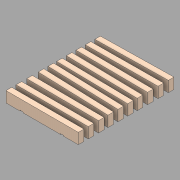
# Autodesk Inventor part: dormente_final
Saved by Autodesk Inventor 2018 (Build 220112000, 112)
## iProperties
Created: 2018-08-09
Part Number: dormente_final
Material: Wood (Birch)
Document SubType Name: Modeling
Designer: flavi
Density: 0.55 g/cm^3
Appearance: Birch - Natural Polished
Mass: 79200 g
Surface Area: 23040 cm^2
Volume: 144000 cm^3
Author: flavi
Autodesk Inventor part; units mm, degrees
ref_plane "YZ Plane" through (0, 0, 0) normal (1, 0, 0) x (0, 1, 0)
ref_plane "XZ Plane" through (0, 0, 0) normal (0, 1, 0) x (-1, 0, 0)
ref_plane "XY Plane" through (0, 0, 0) normal (0, 0, 1) x (1, 0, 0)
sketch "Sketch5" plane through (0, 0, 0) normal (0, 0, 1) x (1, 0, 0)
  line L0 (-20730, -264417.3398) -> (-20730, -262313.5359)
  line L1 (-20730, -260695.3081) -> (-20730, -258591.5042)
  line L2 (-20730, -256710.4016) -> (-20730, -254606.5977)
  line L3 (-20730, -252422.8748) -> (-20730, -250319.0709)
  line L4 (-20730, -248750.3548) -> (-20730, -246646.5509)
  line L5 (-20730, -241909.1189) -> (-20730, -239805.315)
  line L6 (-20730, -238349.0223) -> (-20730, -236245.2184)
  line L7 (-20730, -234866.3859) -> (-20730, -232762.582)
  line L8 (-20730, -231302.8852) -> (-20730, -229199.0813)
  line L9 (-20730, -243453.9106) -> (-20730, -245557.7145)
  line L10 (6242.9418, -264417.3398) -> (6242.9418, -262313.5359)
  line L11 (6242.9412, -260720.3148) -> (6242.9412, -258616.5109)
  line L12 (6242.9412, -256890.9666) -> (6242.9412, -254787.1627)
  line L13 (6242.9412, -253363.9723) -> (6242.9412, -251260.1684)
  line L14 (6242.9412, -249623.3537) -> (6242.9412, -247519.5498)
  line L15 (6242.9412, -246003.92) -> (6242.9412, -243900.1161)
  line L16 (6242.9412, -242439.6002) -> (6242.9412, -240335.7963)
  line L17 (6242.9412, -238586.3047) -> (6242.9412, -236482.5008)
  line L18 (6242.9412, -234655.2907) -> (6242.9412, -232551.4868)
  line L19 (6242.9412, -230805.0616) -> (6242.9412, -228701.2577)
  line L20 (6242.9418, -264417.3398) -> (-20730, -264417.3398)
  line L21 (-20730, -262313.5359) -> (6242.9418, -262313.5359)
  line L22 (6242.9412, -260720.3148) -> (-20730, -260695.3081)
  line L23 (-20730, -258591.5042) -> (6242.9412, -258616.5109)
  line L24 (6242.9412, -256890.9666) -> (-20730, -256710.4016)
  line L25 (-20730, -254606.5977) -> (6242.9412, -254787.1627)
  line L26 (6242.9412, -253363.9723) -> (-20730, -252422.8748)
  line L27 (-20730, -250319.0709) -> (6242.9412, -251260.1684)
  line L28 (6242.9412, -249623.3537) -> (-20730, -248750.3548)
  line L29 (-20730, -246646.5509) -> (6242.9412, -247519.5498)
  line L30 (6242.9412, -246003.92) -> (-20730, -245557.7145)
  line L31 (-20730, -243453.9106) -> (6242.9412, -243900.1161)
  line L32 (-20730, -241909.1189) -> (6242.9412, -242439.6002)
  line L33 (6242.9412, -240335.7963) -> (-20730, -239805.315)
  line L34 (-20730, -238349.0223) -> (6242.9412, -238586.3047)
  line L35 (6242.9412, -236482.5008) -> (-20730, -236245.2184)
  line L36 (-20730, -234866.3859) -> (6242.9412, -234655.2907)
  line L37 (6242.9412, -232551.4868) -> (-20730, -232762.582)
  line L38 (-20730, -231302.8852) -> (6242.9412, -230805.0616)
  line L39 (6242.9412, -228701.2577) -> (-20730, -229199.0813)
  point P0 (0, 0)
  point P1 (-20967.6471, -21622.2237)
  point P2 (6005.2941, -22128.6389)
  point P3 (-20967.6471, -23726.0276)
  point P4 (6005.2941, -24232.4428)
  point P5 (-20967.6471, -25741.5078)
  point P6 (6005.2941, -26024.2617)
  point P7 (-20967.6471, -27845.3117)
  point P8 (6005.2941, -28128.0656)
  point P9 (-20967.6471, -29322.81)
  point P10 (6005.2941, -29455.9796)
  point P11 (-20967.6471, -31426.6139)
  point P12 (6005.2941, -31559.7835)
  point P13 (-20967.6471, -32751.5457)
  point P14 (6005.2941, -33039.4294)
  point P15 (-20967.6471, -34855.3496)
  point P16 (6005.2941, -35143.2333)
  point P17 (-20967.6471, -36586.2217)
  point P18 (6005.2941, -36019.7541)
  point P19 (-20967.6471, -38690.0256)
  point P20 (6005.2941, -38123.558)
  point P21 (-20967.6471, -40394.1013)
  point P22 (6005.2941, -39825.798)
  point P23 (-20967.6471, -42497.9052)
  point P24 (6005.2941, -41929.6019)
  point P25 (-20967.6471, -44164.6545)
  point P26 (6005.2941, -43868.5054)
  point P27 (-20967.6471, -46268.4584)
  point P28 (6005.2941, -45972.3094)
  point P29 (-20967.6471, -47624.7575)
  point P30 (6124.1176, -47419.887)
  point P31 (-20967.6471, -49728.5614)
  point P32 (6124.1176, -49523.6909)
  point P33 (-20967.6471, -51405.068)
  point P34 (6124.1176, -50852.6184)
  point P35 (-20967.6471, -53508.8719)
  point P36 (6124.1176, -52956.4223)
  point P37 (-20967.6471, -58361.4939)
  point P38 (6124.1176, -57120.5712)
  point P39 (-20967.6471, -60465.2978)
  point P40 (6124.1176, -59224.3751)
  point P41 (-20967.6471, -60920.5609)
  point P42 (6124.1176, -60371.9053)
  point P43 (-20967.6471, -63024.3648)
  point P44 (6124.1176, -62475.7093)
  point P45 (-20848.8235, -64155.5217)
  point P46 (6124.1176, -64350.4137)
  point P47 (-20848.8235, -66259.3256)
  point P48 (6124.1176, -66454.2176)
  point P49 (-20848.8235, -67844.0876)
  point P50 (6124.1176, -68075.3244)
  point P51 (-20848.8235, -69947.8915)
  point P52 (6124.1176, -70179.1283)
  point P53 (-20848.8235, -71566.6692)
  point P54 (6124.1176, -71765.9876)
  point P55 (-20848.8235, -73670.4731)
  point P56 (6124.1176, -73869.7915)
  point P57 (-20848.8235, -75189.4885)
  point P58 (6124.1176, -75557.0021)
  point P59 (-20848.8235, -77293.2924)
  point P60 (6124.1176, -77660.806)
  point P61 (-20848.8235, -78800.4247)
  point P62 (6124.1176, -79158.9919)
  point P63 (-20848.8235, -80904.2286)
  point P64 (6124.1176, -81262.7958)
  point P65 (-20848.8235, -82340.3345)
  point P66 (6124.1176, -82631.5147)
  point P67 (-20848.8235, -84444.1384)
  point P68 (6124.1176, -84735.3186)
  point P69 (-20848.8235, -86304.7162)
  point P70 (6124.1176, -85878.5865)
  point P71 (-20848.8235, -88408.5201)
  point P72 (6124.1176, -87982.3904)
  point P73 (-20848.8235, -89831.6613)
  point P74 (6124.1176, -90167.2876)
  point P75 (-20848.8235, -91935.4652)
  point P76 (6124.1176, -92271.0915)
  point P77 (-20848.8235, -93513.8337)
  point P78 (6124.1176, -93898.5101)
  point P79 (-20848.8235, -95617.6376)
  point P80 (6124.1176, -96002.314)
  point P81 (-20848.8235, -102847.812)
  point P82 (6124.1176, -102395.7335)
  point P83 (-20848.8235, -104951.6159)
  point P84 (6124.1176, -104499.5374)
  point P85 (-20848.8235, -106342.4532)
  point P86 (6124.1176, -106515.4114)
  point P87 (-20848.8235, -108446.2571)
  point P88 (6124.1176, -108619.2153)
  point P89 (-20848.8235, -109981.1716)
  point P90 (6124.1176, -110089.6631)
  point P91 (-20848.8235, -112084.9755)
  point P92 (6124.1176, -112193.467)
  point P93 (-20848.8235, -113751.8742)
  point P94 (6124.1176, -113732.3134)
  point P95 (-20848.8235, -115855.6781)
  point P96 (6124.1176, -115836.1173)
  point P97 (-20848.8235, -117298.3112)
  point P98 (6124.1176, -117799.6039)
  point P99 (-20848.8235, -119402.1151)
  point P100 (6124.1176, -119903.4078)
  point P101 (-20848.8235, -120988.6147)
  point P102 (6124.1176, -121322.2726)
  point P103 (-20848.8235, -123092.4186)
  point P104 (6124.1176, -123426.0765)
  point P105 (-20848.8235, -124104.6291)
  point P106 (6124.1176, -124617.6757)
  point P107 (-20848.8235, -126208.433)
  point P108 (6124.1176, -126721.4796)
  point P109 (-20848.8235, -127960.9362)
  point P110 (6124.1176, -128375.0805)
  point P111 (-20848.8235, -130064.7401)
  point P112 (6124.1176, -130478.8844)
  point P113 (-20848.8235, -132255.5715)
  point P114 (6124.1176, -132095.4557)
  point P115 (-20848.8235, -134359.3754)
  point P116 (6124.1176, -134199.2597)
  point P117 (-20848.8235, -135675.5926)
  point P118 (6124.1176, -135487.8273)
  point P119 (-20848.8235, -137779.3965)
  point P120 (6124.1176, -137591.6312)
  point P121 (-20848.8235, -144607.9861)
  point P122 (6124.1176, -144387.8571)
  point P123 (-20848.8235, -146711.79)
  point P124 (6124.1176, -146491.661)
  point P125 (-20848.8235, -148314.0751)
  point P126 (6124.1176, -148295.1438)
  point P127 (-20848.8235, -150417.879)
  point P128 (6124.1176, -150398.9477)
  point P129 (-20848.8235, -152139.9424)
  point P130 (6124.1176, -152482.8636)
  point P131 (-20848.8235, -154243.7463)
  point P132 (6124.1176, -154586.6675)
  point P133 (-20848.8235, -155757.3569)
  point P134 (6124.1176, -156278.2711)
  point P135 (-20848.8235, -157861.1608)
  point P136 (6124.1176, -158382.075)
  point P137 (-20848.8235, -159323.05)
  point P138 (6124.1176, -159925.243)
  point P139 (-20848.8235, -161426.8539)
  point P140 (6124.1176, -162029.0469)
  point P141 (-20848.8235, -162986.1529)
  point P142 (6124.1176, -163475.4003)
  point P143 (-20848.8235, -165089.9568)
  point P144 (6124.1176, -165579.2042)
  point P145 (-20848.8235, -166721.6427)
  point P146 (6124.1176, -167153.3914)
  point P147 (-20848.8235, -168825.4466)
  point P148 (6124.1176, -169257.1953)
  point P149 (-20848.8235, -170217.6991)
  point P150 (6242.9412, -170671.8236)
  point P151 (-20848.8235, -172321.503)
  point P152 (6242.9412, -172775.6275)
  point P153 (-20848.8235, -174234.1043)
  point P154 (6242.9412, -174268.9144)
  point P155 (-20848.8235, -176337.9082)
  point P156 (6242.9412, -176372.7184)
  point P157 (-20848.8235, -178049.9898)
  point P158 (6242.9412, -177866.4022)
  point P159 (-20848.8235, -180153.7937)
  point P160 (6242.9412, -179970.2061)
  point P161 (-20848.8235, -186925.1382)
  point P162 (6242.9412, -187023.8253)
  point P163 (-20848.8235, -189028.9421)
  point P164 (6242.9412, -189127.6292)
  point P165 (-20730, -190608.4103)
  point P166 (6242.9412, -190955.6253)
  point P167 (-20730, -192712.2142)
  point P168 (6242.9412, -193059.4292)
  point P169 (-20730, -194360.1448)
  point P170 (6242.9412, -194817.9349)
  point P171 (-20730, -196463.9487)
  point P172 (6242.9412, -196921.7388)
  point P173 (-20730, -198017.5791)
  point P174 (6242.9412, -198574.0909)
  point P175 (-20730, -200121.383)
  point P176 (6242.9412, -200677.8948)
  point P177 (-20730, -201788.5309)
  point P178 (6242.9412, -202216.0346)
  point P179 (-20730, -203892.3348)
  point P180 (6242.9412, -204319.8385)
  point P181 (-20730, -205635.6546)
  point P182 (6242.9412, -205781.4811)
  point P183 (-20730, -207739.4585)
  point P184 (6242.9412, -207885.285)
  point P185 (-20730, -209497.3663)
  point P186 (6242.9412, -209131.5896)
  point P187 (-20730, -211601.1702)
  point P188 (6242.9412, -211235.3935)
  point P189 (-20730, -213181.738)
  point P190 (6242.9412, -212258.4637)
  point P191 (-20730, -215285.5419)
  point P192 (6242.9412, -214362.2676)
  point P193 (-20730, -216668.1961)
  point P194 (6242.9412, -215985.7199)
  point P195 (-20730, -218772)
  point P196 (6242.9412, -218089.5238)
  point P197 (-20730, -220095.541)
  point P198 (6242.9412, -219772.1543)
  point P199 (-20730, -222199.3449)
  constraints: 80 end point, 10 parallel, 3 vertical, 1 horizontal
sketch "Sketch6" plane through (0, 0, 0) normal (0, 0, 1) x (1, 0, 0)
  line L0 (-411.1765, -264436.5073) -> (-411.1765, -262309.305)
  line L1 (-411.1765, -262309.305) -> (-411.1765, -260714.1457)
  line L2 (-411.1765, -260714.1457) -> (-411.1765, -258610.3418)
  line L3 (-411.1765, -258610.3418) -> (-411.1765, -256846.4219)
  line L4 (-411.1765, -256846.4219) -> (-411.1765, -254742.618)
  line L5 (-411.1765, -254742.618) -> (-292.3529, -253135.9531)
  line L6 (-292.3529, -253135.9531) -> (-292.3529, -251032.1492)
  line L7 (-292.3529, -251032.1492) -> (-292.3529, -249411.8341)
  line L8 (-292.3529, -249411.8341) -> (-292.3529, -247308.0302)
  line L9 (-292.3529, -247308.0302) -> (-292.3529, -245895.8085)
  line L10 (-292.3529, -245895.8085) -> (-292.3529, -243792.0046)
  line L11 (-292.3529, -243792.0046) -> (-411.1765, -242308.7326)
  line L12 (-411.1765, -242308.7326) -> (-411.1765, -240204.9286)
  line L13 (-411.1765, -240204.9286) -> (-411.1765, -238527.7681)
  line L14 (-411.1765, -238527.7681) -> (-411.1765, -236423.9642)
  line L15 (-411.1765, -236423.9642) -> (-411.1765, -234707.3671)
  line L16 (-411.1765, -234707.3671) -> (-411.1765, -232603.5631)
  line L17 (-411.1765, -232603.5631) -> (-287.1139, -230926.0589)
  line L18 (-287.1139, -230926.0589) -> (-287.1139, -228740.268)
  line L19 (-287.1139, -228740.268) -> (777.2418, -228740.268)
  line L20 (777.2418, -228740.268) -> (777.2418, -230906.1896)
  line L21 (777.2418, -230906.1896) -> (777.2418, -232594.5112)
  line L22 (777.2418, -232594.5112) -> (777.2418, -234698.3151)
  line L23 (777.2418, -234698.3151) -> (777.2418, -236434.6646)
  line L24 (777.2418, -236434.6646) -> (777.2418, -238538.4685)
  line L25 (777.2418, -238538.4685) -> (777.2418, -240228.5453)
  line L26 (777.2418, -240228.5453) -> (777.2418, -242332.3492)
  line L27 (777.2418, -242332.3492) -> (777.2418, -243809.943)
  line L28 (777.2418, -243809.943) -> (777.2418, -245913.7469)
  line L29 (777.2418, -245913.7469) -> (777.2418, -247342.8899)
  line L30 (777.2418, -247342.8899) -> (777.2418, -249446.6938)
  line L31 (777.2418, -249446.6938) -> (777.2418, -251069.7089)
  line L32 (777.2418, -251069.7089) -> (777.2418, -253173.5128)
  line L33 (777.2418, -253173.5128) -> (777.2418, -254750.8199)
  line L34 (777.2418, -254750.8199) -> (777.2418, -256854.6238)
  line L35 (777.2418, -256854.6238) -> (777.2418, -258611.6909)
  line L36 (777.2418, -258611.6909) -> (777.2418, -260715.4948)
  line L37 (777.2418, -260715.4948) -> (777.2418, -262309.305)
  line L38 (777.2418, -262309.305) -> (777.2418, -264436.5073)
  line L39 (777.2418, -264436.5073) -> (-411.1765, -264436.5073)
  line L40 (-14313.5294, -264431.9833) -> (-14313.5294, -262312.3235)
  line L41 (-14313.5294, -262312.3235) -> (-14313.5294, -260701.3806)
  line L42 (-14313.5294, -260701.3806) -> (-14313.5294, -258597.5767)
  line L43 (-14313.5294, -258597.5767) -> (-14313.5294, -256753.4791)
  line L44 (-14313.5294, -256753.4791) -> (-14313.5294, -254649.6752)
  line L45 (-14313.5294, -254649.6752) -> (-14313.5294, -252646.872)
  line L46 (-14313.5294, -252646.872) -> (-14313.5294, -250543.068)
  line L47 (-14313.5294, -250543.068) -> (-14313.5294, -248958.1522)
  line L48 (-14313.5294, -248958.1522) -> (-14313.5294, -246854.3483)
  line L49 (-14313.5294, -246854.3483) -> (-14313.5294, -245663.984)
  line L50 (-14313.5294, -245663.984) -> (-14313.5294, -243560.1801)
  line L51 (-14313.5294, -243560.1801) -> (-14313.5294, -229054.1614)
  line L52 (-14313.5294, -229054.1614) -> (-15501.7647, -229075.8446)
  line L53 (-15501.7647, -229075.8446) -> (-15501.7647, -231206.2671)
  line L54 (-15501.7647, -231206.2671) -> (-15501.7647, -232721.5412)
  line L55 (-15501.7647, -232721.5412) -> (-15501.7647, -260700.0315)
  line L56 (-15501.7647, -260700.0315) -> (-15501.7647, -262312.3235)
  line L57 (-15501.7647, -262312.3235) -> (-15501.7647, -264431.9833)
  line L58 (-15501.7647, -264431.9833) -> (-14313.5294, -264431.9833)
  point P0 (0, 0)
  point P1 (-15739.4118, -21720.3835)
  point P2 (-14551.1765, -21742.6925)
  point P3 (-411.1765, -22008.1701)
  point P4 (777.0588, -22030.4791)
  point P5 (-15739.4118, -23824.1874)
  point P6 (-14551.1765, -23846.4964)
  point P7 (-411.1765, -24111.974)
  point P8 (777.0588, -24134.283)
  point P9 (-15739.4118, -25796.3147)
  point P10 (-14551.1765, -25808.7709)
  point P11 (-411.1765, -25956.9987)
  point P12 (777.0588, -25969.4548)
  point P13 (-15739.4118, -27900.1186)
  point P14 (-14551.1765, -27912.5748)
  point P15 (-411.1765, -28060.8026)
  point P16 (777.0588, -28073.2587)
  point P17 (-15739.4118, -29348.6226)
  point P18 (-14551.1765, -29354.4891)
  point P19 (-411.1765, -29424.3005)
  point P20 (777.0588, -29430.167)
  point P21 (-15739.4118, -31452.4265)
  point P22 (-14551.1765, -31458.293)
  point P23 (-411.1765, -31528.1044)
  point P24 (777.0588, -31533.9709)
  point P25 (-15739.4118, -32807.347)
  point P26 (-14551.1765, -32820.0291)
  point P27 (-411.1765, -32970.9461)
  point P28 (777.0588, -32983.6282)
  point P29 (-15739.4118, -34911.1509)
  point P30 (-14551.1765, -34923.833)
  point P31 (-411.1765, -35074.75)
  point P32 (777.0588, -35087.4321)
  point P33 (-15739.4118, -36476.4218)
  point P34 (-14551.1765, -36451.4673)
  point P35 (-411.1765, -36154.5085)
  point P36 (777.0588, -36129.554)
  point P37 (-15739.4118, -38580.2257)
  point P38 (-14551.1765, -38555.2712)
  point P39 (-411.1765, -38258.3124)
  point P40 (777.0588, -38233.3579)
  point P41 (-15739.4118, -40283.9456)
  point P42 (-14551.1765, -40258.9102)
  point P43 (-411.1765, -39960.9891)
  point P44 (777.0588, -39935.9537)
  point P45 (-15739.4118, -42387.7495)
  point P46 (-14551.1765, -42362.7141)
  point P47 (-411.1765, -42064.793)
  point P48 (777.0588, -42039.7576)
  point P49 (-15739.4118, -44107.2512)
  point P50 (-14551.1765, -44094.205)
  point P51 (-411.1765, -43938.955)
  point P52 (777.0588, -43925.9088)
  point P53 (-15739.4118, -46211.0551)
  point P54 (-14551.1765, -46198.0089)
  point P55 (-411.1765, -46042.7589)
  point P56 (777.0588, -46029.7127)
  point P57 (-15739.4118, -47585.2211)
  point P58 (-14551.1765, -47576.2356)
  point P59 (-411.1765, -47469.3075)
  point P60 (777.0588, -47460.3219)
  point P61 (-15739.4118, -49689.025)
  point P62 (-14551.1765, -49680.0395)
  point P63 (-411.1765, -49573.1114)
  point P64 (777.0588, -49564.1259)
  point P65 (-15739.4118, -51298.4549)
  point P66 (-14551.1765, -51274.2246)
  point P67 (-411.1765, -50985.8847)
  point P68 (777.0588, -50961.6545)
  point P69 (-15739.4118, -53402.2588)
  point P70 (-14551.1765, -53378.0285)
  point P71 (-411.1765, -53089.6886)
  point P72 (777.0588, -53065.4584)
  point P73 (-15739.4118, -58122.0176)
  point P74 (-14551.1765, -58067.5912)
  point P75 (-292.3529, -57414.4739)
  point P76 (777.0588, -57365.4901)
  point P77 (-15739.4118, -60225.8215)
  point P78 (-14551.1765, -60171.3951)
  point P79 (-292.3529, -59518.2778)
  point P80 (777.0588, -59469.294)
  point P81 (-15739.4118, -60814.68)
  point P82 (-14551.1765, -60790.6162)
  point P83 (-411.1765, -60504.2565)
  point P84 (777.0588, -60480.1926)
  point P85 (-15739.4118, -62918.4839)
  point P86 (-14551.1765, -62894.4201)
  point P87 (-411.1765, -62608.0604)
  point P88 (777.0588, -62583.9965)
  point P89 (-15739.4118, -64192.4395)
  point P90 (-14551.1765, -64201.0251)
  point P91 (-411.1765, -64303.1932)
  point P92 (777.0588, -64311.7787)
  point P93 (-15739.4118, -66296.2434)
  point P94 (-14551.1765, -66304.829)
  point P95 (-411.1765, -66406.9971)
  point P96 (777.0588, -66415.5826)
  point P97 (-15739.4118, -67887.8901)
  point P98 (-14551.1765, -67898.0768)
  point P99 (-411.1765, -68019.2978)
  point P100 (777.0588, -68029.4845)
  point P101 (-15739.4118, -69991.6941)
  point P102 (-14551.1765, -70001.8807)
  point P103 (-411.1765, -70123.1017)
  point P104 (777.0588, -70133.2884)
  point P105 (-15739.4118, -71604.4255)
  point P106 (-14551.1765, -71613.2061)
  point P107 (-411.1765, -71717.6946)
  point P108 (777.0588, -71726.4751)
  point P109 (-15739.4118, -73708.2295)
  point P110 (-14551.1765, -73717.01)
  point P111 (-411.1765, -73821.4985)
  point P112 (777.0588, -73830.279)
  point P113 (-15739.4118, -75259.1056)
  point P114 (-14551.1765, -75275.2956)
  point P115 (-411.1765, -75467.9569)
  point P116 (777.0588, -75484.147)
  point P117 (-15739.4118, -77362.9095)
  point P118 (-14551.1765, -77379.0995)
  point P119 (-411.1765, -77571.7609)
  point P120 (777.0588, -77587.9509)
  point P121 (-15739.4118, -78868.3471)
  point P122 (-14551.1765, -78884.143)
  point P123 (-411.1765, -79072.1144)
  point P124 (777.0588, -79087.9103)
  point P125 (-15739.4118, -80972.151)
  point P126 (-14551.1765, -80987.9469)
  point P127 (-411.1765, -81175.9183)
  point P128 (777.0588, -81191.7142)
  point P129 (-15739.4118, -82395.492)
  point P130 (-14551.1765, -82408.3193)
  point P131 (-411.1765, -82560.9644)
  point P132 (777.0588, -82573.7917)
  point P133 (-15739.4118, -84499.2959)
  point P134 (-14551.1765, -84512.1232)
  point P135 (-411.1765, -84664.7683)
  point P136 (777.0588, -84677.5956)
  point P137 (-15739.4118, -86223.9956)
  point P138 (-14551.1765, -86205.2234)
  point P139 (-411.1765, -85981.8338)
  point P140 (777.0588, -85963.0616)
  point P141 (-15739.4118, -88327.7995)
  point P142 (-14551.1765, -88309.0273)
  point P143 (-411.1765, -88085.6377)
  point P144 (777.0588, -88066.8655)
  point P145 (-15739.4118, -89895.2381)
  point P146 (-14432.3529, -89911.5019)
  point P147 (-411.1765, -90085.9685)
  point P148 (777.0588, -90100.7538)
  point P149 (-15620.5882, -92000.5205)
  point P150 (-14432.3529, -92015.3058)
  point P151 (-411.1765, -92189.7724)
  point P152 (777.0588, -92204.5577)
  point P153 (-15620.5882, -93588.3965)
  point P154 (-14432.3529, -93605.3426)
  point P155 (-411.1765, -93805.3066)
  point P156 (777.0588, -93822.2526)
  point P157 (-15620.5882, -95692.2004)
  point P158 (-14432.3529, -95709.1465)
  point P159 (-411.1765, -95909.1105)
  point P160 (777.0588, -95926.0566)
  point P161 (-15620.5882, -102760.1844)
  point P162 (-14432.3529, -102740.2691)
  point P163 (-411.1765, -102505.268)
  point P164 (777.0588, -102485.3526)
  point P165 (-15620.5882, -104863.9883)
  point P166 (-14432.3529, -104844.073)
  point P167 (-411.1765, -104609.0719)
  point P168 (777.0588, -104589.1565)
  point P169 (-15620.5882, -106375.9782)
  point P170 (-14432.3529, -106383.5975)
  point P171 (-411.1765, -106473.5052)
  point P172 (777.0588, -106481.1245)
  point P173 (-15620.5882, -108479.7821)
  point P174 (-14432.3529, -108487.4014)
  point P175 (-411.1765, -108577.3091)
  point P176 (777.0588, -108584.9284)
  point P177 (-15620.5882, -110002.2008)
  point P178 (-14432.3529, -110006.9801)
  point P179 (-411.1765, -110063.3766)
  point P180 (777.0588, -110068.1559)
  point P181 (-15620.5882, -112106.0047)
  point P182 (-14432.3529, -112110.784)
  point P183 (-411.1765, -112167.1805)
  point P184 (777.0588, -112171.9599)
  point P185 (-15620.5882, -113748.0827)
  point P186 (-14432.3529, -113747.221)
  point P187 (-411.1765, -113737.0528)
  point P188 (777.0588, -113736.1911)
  point P189 (-15620.5882, -115851.8866)
  point P190 (-14432.3529, -115851.0249)
  point P191 (-411.1765, -115840.8567)
  point P192 (777.0588, -115839.995)
  point P193 (-15620.5882, -117395.478)
  point P194 (-14432.3529, -117417.5614)
  point P195 (-411.1765, -117678.1453)
  point P196 (777.0588, -117700.2287)
  point P197 (-15620.5882, -119499.2819)
  point P198 (-14432.3529, -119521.3653)
  point P199 (-411.1765, -119781.9492)
  constraints: 118 end point, 46 collinear, 4 parallel, 4 perpendicular, 2 vertical
sketch "Sketch7" plane through (0, 0, 0) normal (0, 0, 1) x (1, 0, 0)
  line L0 (-14313.5294, -243560.1801) -> (-14313.5294, -229054.1614) projected
  line L1 (-287.1139, -230926.0589) -> (-287.1139, -228740.268) projected
  line L2 (-411.1765, -232603.5631) -> (-287.1139, -230926.0589) projected
  line L3 (-411.1765, -238527.7681) -> (-411.1765, -236423.9642) projected
  line L4 (-411.1765, -240204.9286) -> (-411.1765, -238527.7681) projected
  line L5 (-411.1765, -242308.7326) -> (-411.1765, -240204.9286) projected
  line L6 (-292.3529, -243792.0046) -> (-411.1765, -242308.7326) projected
  line L7 (-292.3529, -245895.8085) -> (-292.3529, -243792.0046) projected
  line L8 (-292.3529, -247308.0302) -> (-292.3529, -245895.8085) projected
  line L9 (-292.3529, -249411.8341) -> (-292.3529, -247308.0302) projected
  line L10 (-292.3529, -251032.1492) -> (-292.3529, -249411.8341) projected
  line L11 (-292.3529, -253135.9531) -> (-292.3529, -251032.1492) projected
  line L12 (-411.1765, -254742.618) -> (-292.3529, -253135.9531) projected
  line L13 (-411.1765, -256846.4219) -> (-411.1765, -254742.618) projected
  line L14 (-411.1765, -258610.3418) -> (-411.1765, -256846.4219) projected
  line L15 (-411.1765, -260714.1457) -> (-411.1765, -258610.3418) projected
  line L16 (-411.1765, -262309.305) -> (-411.1765, -260714.1457) projected
  line L17 (-411.1765, -264436.5073) -> (-411.1765, -262309.305) projected
  line L18 (-14313.5294, -264431.9833) -> (-14313.5294, -262312.3235) projected
  line L19 (-14313.5294, -262312.3235) -> (-14313.5294, -260701.3806) projected
  line L20 (-14313.5294, -260701.3806) -> (-14313.5294, -258597.5767) projected
  line L21 (-14313.5294, -258597.5767) -> (-14313.5294, -256753.4791) projected
  line L22 (-14313.5294, -256753.4791) -> (-14313.5294, -254649.6752) projected
  line L23 (-14313.5294, -254649.6752) -> (-14313.5294, -252646.872) projected
  line L24 (-14313.5294, -252646.872) -> (-14313.5294, -250543.068) projected
  line L25 (-14313.5294, -250543.068) -> (-14313.5294, -248958.1522) projected
  line L26 (-14313.5294, -248958.1522) -> (-14313.5294, -246854.3483) projected
  line L27 (-9679.4118, -231098.9311) -> (-8015.8824, -232663.079)
  line L28 (-8015.8824, -232663.079) -> (-5995.8824, -234751.074)
  line L29 (-5995.8824, -234751.074) -> (-4332.3529, -236389.4694)
  line L30 (-4332.3529, -236389.4694) -> (-2185.4671, -238503.9182)
  line L31 (-2185.4671, -238503.9182) -> (-536.6634, -240208.2221)
  line L32 (-536.6634, -240208.2221) -> (-424.8776, -240323.7708)
  line L33 (-3380.4513, -240146.4004) -> (-536.6634, -243002.8524)
  line L34 (-536.6634, -243002.8524) -> (-411.1765, -242308.7326)
  line L35 (-3380.4513, -240146.4004) -> (-5045.2941, -238487.0015)
  line L36 (-5045.2941, -238487.0015) -> (-7184.1176, -236364.3822)
  line L37 (-7184.1176, -236364.3822) -> (-8728.8235, -234772.4625)
  line L38 (-8728.8235, -234772.4625) -> (-10867.647, -232685.3974)
  line L39 (-10867.647, -232685.3974) -> (-12412.3529, -231149.3713)
  line L40 (-12412.3529, -231149.3713) -> (-14313.5294, -229226.0289)
  line L41 (-14313.5294, -229226.0289) -> (-14313.5294, -229063.2452)
  line L42 (-11699.4118, -229032.4091) -> (-14313.5294, -229063.2452)
  line L43 (-11699.4118, -229032.4091) -> (-9679.4118, -231098.9311)
  line L44 (-9798.2353, -258601.6391) -> (-8015.8824, -256795.5137)
  line L45 (-8015.8824, -256795.5137) -> (-5995.8824, -254705.2323)
  line L46 (-5995.8824, -254705.2323) -> (-4332.3529, -252994.9958)
  line L47 (-4332.3529, -252994.9958) -> (-2431.1765, -250957.5247)
  line L48 (-2431.1765, -250957.5247) -> (-886.6651, -249392.4132)
  line L49 (-886.6651, -249392.4132) -> (-411.1765, -248918.6515)
  line L50 (-411.1765, -248918.6515) -> (-292.3529, -248800.2595)
  line L51 (-292.3529, -247178.9498) -> (-1480.5882, -247269.5721)
  line L52 (-1480.5882, -247269.5721) -> (-3496.3345, -249312.2037)
  line L53 (-3496.3345, -249312.2037) -> (-5045.3302, -250866.2811)
  line L54 (-5045.3302, -250866.2811) -> (-6946.5078, -252903.7534)
  line L55 (-6946.5078, -252903.7534) -> (-8728.8235, -254686.9372)
  line L56 (-8728.8235, -254686.9372) -> (-10748.8235, -256777.2186)
  line L57 (-10748.8235, -256777.2186) -> (-12531.1765, -258599.1054)
  line L58 (-12531.1765, -258599.1054) -> (-14313.5294, -260475.0945)
  line L59 (-14313.5294, -260475.0945) -> (-14313.5294, -263280.1663)
  line L60 (-14313.5294, -263280.1663) -> (-13364.6935, -262310.2845)
  line L61 (-13364.6935, -262310.2845) -> (-11815.0088, -260706.682)
  line L62 (-11815.0088, -260706.682) -> (-9798.2353, -258601.6391)
  line L63 (-411.1765, -242308.7326) -> (-411.1765, -242308.7326)
  line L64 (-411.1765, -242308.7326) -> (-411.1765, -240337.933)
  line L65 (-424.8776, -240323.7708) -> (-411.1765, -240337.933)
  point P0 (0, 0)
  point P1 (-6471.1765, -21894.394)
  point P2 (-3381.7647, -21952.3975)
  point P3 (-8847.6471, -23953.5798)
  point P4 (-5758.2353, -24011.5833)
  point P5 (-10867.6471, -25847.3848)
  point P6 (-7778.2353, -25879.7707)
  point P7 (-13244.1176, -27926.2765)
  point P8 (-10154.7059, -27958.6624)
  point P9 (-11699.4118, -29368.5687)
  point P10 (-14075.8824, -31460.6396)
  point P11 (-13006.4706, -38522.8303)
  point P12 (-10748.8235, -40178.797)
  point P13 (-14432.3529, -40256.4067)
  point P14 (-8015.8824, -42225.0195)
  point P15 (-11699.4118, -42302.6292)
  point P16 (-5639.4118, -43996.3583)
  point P17 (-9322.9412, -44036.8016)
  point P18 (-2787.6471, -46068.8513)
  point P19 (-6590, -46110.5992)
  point P20 (-886.4706, -47472.9017)
  point P21 (-4688.8235, -47501.6555)
  point P22 (-1837.0588, -49583.8941)
  point P23 (-14313.5294, -58056.7059)
  point P24 (-12293.5294, -60067.9848)
  point P25 (-11580.5882, -60730.4566)
  point P26 (-14313.5294, -60785.8034)
  point P27 (-9560.5882, -62793.352)
  point P28 (-12293.5294, -62848.6988)
  point P29 (-8015.8824, -64248.2456)
  point P30 (-10867.6471, -64227.6403)
  point P31 (-5877.0588, -66367.5035)
  point P32 (-8728.8235, -66346.8982)
  point P33 (-4332.3529, -67985.6819)
  point P34 (-7184.1176, -67961.234)
  point P35 (-2193.5294, -70107.8218)
  point P36 (-5045.2941, -70083.3738)
  point P37 (-530, -71716.8165)
  point P38 (-3381.7647, -71695.7432)
  point P39 (-1242.9412, -73815.3521)
  point P40 (-1005.2941, -79064.2165)
  point P41 (-3500.5882, -81134.8489)
  point P42 (-5045.2941, -82510.9379)
  point P43 (-1837.0588, -82545.5716)
  point P44 (-7421.7647, -84589.0871)
  point P45 (-4213.5294, -84623.7209)
  point P46 (-9204.1176, -86120.7483)
  point P47 (-5877.0588, -86068.1861)
  point P48 (-11699.4118, -88263.9739)
  point P49 (-8372.3529, -88211.4117)
  point P50 (-13600.5882, -89921.8516)
  point P51 (-10392.3529, -89961.7719)
  point P52 (-12768.8235, -92036.0052)
  point P53 (-3381.7647, -102555.0563)
  point P54 (-5995.8824, -104702.674)
  point P55 (-2431.1765, -104642.928)
  point P56 (-8015.8824, -106424.7417)
  point P57 (-4688.8235, -106446.0757)
  point P58 (-10511.1765, -108512.5451)
  point P59 (-7184.1176, -108533.8791)
  point P60 (-12412.3529, -110015.105)
  point P61 (-8966.4706, -110028.9652)
  point P62 (-11580.5882, -112122.2545)
  point P63 (-13481.7647, -113746.5316)
  point P64 (-12887.6471, -121087.0952)
  point P65 (-10511.1765, -123220.2963)
  point P66 (-13600.5882, -123182.08)
  point P67 (-9204.1176, -124326.1206)
  point P68 (-12412.3529, -124265.0974)
  point P69 (-6827.6471, -126475.1268)
  point P70 (-10035.8824, -126414.1037)
  point P71 (-4926.4706, -128205.409)
  point P72 (-8134.7059, -128156.1496)
  point P73 (-2550, -130345.7014)
  point P74 (-5758.2353, -130296.442)
  point P75 (-530, -132134.9557)
  point P76 (-3619.4118, -132153.2949)
  point P77 (-1361.7647, -134243.6971)
  point P78 (-13006.4706, -144543.9838)
  point P79 (-10511.1765, -146627.4234)
  point P80 (-13957.0588, -146655.5456)
  point P81 (-8372.3529, -148305.3183)
  point P82 (-11937.0588, -148307.8203)
  point P83 (-5877.0588, -150407.3709)
  point P84 (-9322.9412, -150409.7894)
  point P85 (-3381.7647, -152362.0103)
  point P86 (-6946.4706, -152316.6903)
  point P87 (-767.6471, -154499.0488)
  point P88 (-4332.3529, -154453.7289)
  point P89 (-2312.3529, -156115.342)
  point P90 (-1599.4118, -163335.3075)
  point P91 (-3857.0588, -165398.1611)
  point P92 (-886.4706, -165452.043)
  point P93 (-5520.5882, -166966.9977)
  point P94 (-2550, -167014.5471)
  point P95 (-7778.2353, -169034.664)
  point P96 (-4807.6471, -169082.2134)
  point P97 (-9204.1176, -170412.893)
  point P98 (-6233.5294, -170462.6873)
  point P99 (-11461.7647, -172478.8532)
  point P100 (-8491.1765, -172528.6475)
  point P101 (-13362.9412, -174243.7229)
  point P102 (-10392.3529, -174247.5398)
  point P103 (-12650, -176348.4429)
  point P104 (-2312.3529, -186992.661)
  point P105 (-4807.6471, -189087.3753)
  point P106 (-1480.5882, -189099.4947)
  point P107 (-6827.6471, -190787.3714)
  point P108 (-3500.5882, -190830.1996)
  point P109 (-9322.9412, -192859.0541)
  point P110 (-5995.8824, -192901.8823)
  point P111 (-11342.9412, -194519.4638)
  point P112 (-8015.8824, -194575.9313)
  point P113 (-13838.2353, -196580.9171)
  point P114 (-10511.1765, -196637.3846)
  point P115 (-12412.3529, -198189.1907)
  point P116 (-12768.8235, -205678.6959)
  point P117 (-10748.8235, -207793.4207)
  point P118 (-13481.7647, -207778.6454)
  point P119 (-9204.1176, -209341.0652)
  point P120 (-11937.0588, -209378.1263)
  point P121 (-7302.9412, -211419.0875)
  point P122 (-9917.0588, -211454.5373)
  point P123 (-5995.8824, -212677.3943)
  point P124 (-8610, -212766.8746)
  point P125 (-4094.7059, -214716.1216)
  point P126 (-6708.8235, -214805.6019)
  point P127 (-2668.8235, -216211.2076)
  point P128 (-5282.9412, -216277.3507)
  point P129 (-648.8235, -218263.901)
  point P130 (-3262.9412, -218330.044)
  point P131 (-1837.0588, -219869.0278)
  point P132 (-14432.3529, -37470.0336)
  point P133 (-14432.3529, -37470.0336)
  point P134 (-411.1765, -47836.4535)
  point P135 (-411.1765, -47836.4535)
  point P136 (-411.1765, -71845.8163)
  point P137 (-411.1765, -71845.8163)
  point P138 (-14432.3529, -90653.4022)
  point P139 (-14432.3529, -90653.4022)
  point P140 (-411.1765, -102944.2892)
  point P141 (-411.1765, -102944.2892)
  point P142 (-14432.3529, -111696.0301)
  point P143 (-14432.3529, -111696.0301)
  point P144 (-14432.3529, -114501.1019)
  point P145 (-14432.3529, -114501.1019)
  point P146 (-14432.3529, -122453.2439)
  point P147 (-14432.3529, -122453.2439)
  point P148 (-411.1765, -132278.698)
  point P149 (-411.1765, -132278.698)
  point P150 (-14432.3529, -146238.7136)
  point P151 (-14432.3529, -146238.7136)
  point P152 (-411.1765, -157619.6296)
  point P153 (-411.1765, -157619.6296)
  point P154 (-411.1765, -165066.5592)
  point P155 (-411.1765, -165066.5592)
  point P156 (-14313.5294, -175081.6681)
  point P157 (-14313.5294, -175081.6681)
  point P158 (-411.1765, -188213.1807)
  point P159 (-411.1765, -188213.1807)
  point P160 (-14313.5294, -199777.6558)
  point P161 (-14313.5294, -199777.6558)
  point P162 (-14313.5294, -206905.1589)
  point P163 (-14313.5294, -206905.1589)
  point P164 (-411.1765, -221301.4459)
  point P165 (-411.1765, -221301.4459)
  point P166 (-14313.5294, -229226.0289)
  point P167 (-411.1765, -240309.6776)
  point P168 (-411.1765, -248918.6299)
  point P169 (-411.1765, -248918.6299)
  point P170 (-411.1765, -234707.3671)
  constraints: 78 end point, 8 parallel, 5 point on line, 2 collinear, 1 perpendicular, 1 vertical, 2 other
extrude "Extrusion6" add sketch "Sketch5" along normal blind 4000
extrude "Extrusion7" cut sketch "Sketch6" along normal blind 250
extrude "Extrusion8" cut sketch "Sketch7" along normal blind 500
sketch "Sketch8" plane through (0, 0, 4000) normal (0, 0, 1) x (1, 0, 0)
  line L0 (6242.9412, -238586.3047) -> (6242.9412, -236482.5008) projected
  line L1 (-20730, -236245.2184) -> (-20730, -238349.0223) projected
  line L2 (6242.9412, -236482.5008) -> (-20730, -236245.2184) projected
  line L3 (-20730, -238349.0223) -> (6242.9412, -238586.3047) projected
  line L4 (-20730, -234866.3859) -> (6242.9412, -234655.2907) projected
  point P0 (0, 0)
  dimension "d27" = 26972.9
  dimension "d28" = 2103.7225
  dimension "d29" = 1827.1541
  measures "d27" distance between parallel lines of L0 L1
  measures "d28" distance between parallel lines of L2 L3
  measures "d29" distance from line of L0.end L4
body "Solid4"
